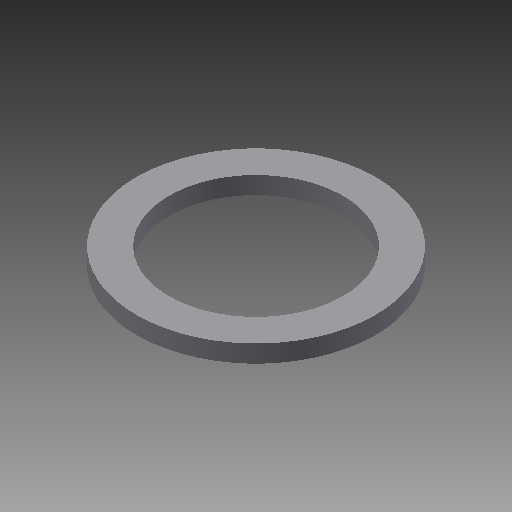
# Autodesk Inventor part: Rondella
Saved by Autodesk Inventor 2019 (Build 230136000, 136)
## iProperties
Created: 2011-10-08
Part Number: Rondella
Document SubType Name: Modeling
Designer: Stefano
Density: 1 g/cm^3
Material: 一般
Appearance: 既定
Author: Stefano
Autodesk Inventor part; units mm, degrees
ref_plane "YZ Plane" through (0, 0, 0) normal (1, 0, 0) x (0, 1, 0)
ref_plane "XZ Plane" through (0, 0, 0) normal (0, 1, 0) x (-1, 0, 0)
ref_plane "XY Plane" through (0, 0, 0) normal (0, 0, 1) x (1, 0, 0)
sketch "Schizzo1" plane through (0, 0, 0) normal (0, 0, 1) x (1, 0, 0)
  line L0 (4, 0) -> (5.5, 0)
  line L1 (5.5, 0) -> (5.5, 0.8)
  line L2 (5.5, 0.8) -> (4, 0.8)
  line L3 (4, 0.8) -> (4, 0)
  line L4 (0, -0.16) -> (0, 0.96) projected
  point P0 (0, 0)
  dimension "d0" = 4
  dimension "d1" = 0.8
  dimension "d2" = 5.5
  constraints: 8 end point, 2 parallel, 1 horizontal, 1 perpendicular
  measures "d0" distance of point (0, 0) L0.start
  measures "d1" distance of L2.end L0.start
  measures "d2" distance from line of L1 point (0, 0)
revolve "Rivoluzione1" add sketch "Schizzo1" angle 360 about axis through (0, -10, 0) along (0, 1, 0)
